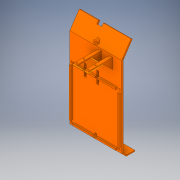
# Autodesk Inventor part: chassis-akksi-top
Saved by Autodesk Inventor 2019 (Build 230136000, 136)
## iProperties
Created: 2019-02-14
Part Number: chassis-akksi-top
Material: Generic
Document SubType Name: Modeling
Designer: izsoandras
Density: 1 g/cm^3
Appearance: Default
Author: izsoandras
Autodesk Inventor part; units mm, degrees
ref_plane "YZ Plane" through (0, 0, 0) normal (1, 0, 0) x (0, 1, 0)
ref_plane "XZ Plane" through (0, 0, 0) normal (0, 1, 0) x (-1, 0, 0)
ref_plane "XY Plane" through (0, 0, 0) normal (0, 0, 1) x (1, 0, 0)
sketch "Sketch1" plane through (0, 0, 0) normal (0, 0, 1) x (1, 0, 0)
  line L0 (59, 131.5) -> (-36.0094, 131.5)
  line L1 (-36.0094, 131.5) -> (-36.0094, -49.2144)
  line L2 (-36.0094, -49.2144) -> (59, -49.2144)
  line L3 (59, -49.2144) -> (59, 131.5)
  point P0 (0, 0)
  point P1 (-36, 131.5)
  point P2 (59.0094, -49.2144)
  constraints: 8 end point, 2 parallel, 1 horizontal, 1 perpendicular, 4 other
extrude "Extrusion1" add sketch "Sketch1" along normal blind 3
sketch "Sketch2" plane through (0, 0, 3) normal (0, 0, 1) x (1, 0, 0)
  line L0 (16.62, 69.08) -> (14.03, 69.08)
  line L1 (14.03, 69.08) -> (14.03, 48.08)
  line L2 (14.03, 48.08) -> (16.62, 48.08)
  line L3 (16.62, 48.08) -> (16.62, 69.08)
  line L4 (-6.41, 48.08) -> (-6.41, 69.08)
  line L5 (-6.41, 69.08) -> (-9, 69.08)
  line L6 (-9, 69.08) -> (-9, 48.08)
  line L7 (-9, 48.08) -> (-6.41, 48.08)
  line L8 (59, 131.5) -> (-36.0094, 131.5)
  line L9 (-36.0094, 131.5) -> (-36.0094, -49.2144)
  line L10 (-36.0094, -49.2144) -> (59, -49.2144)
  line L11 (59, -49.2144) -> (59, 131.5)
  line L12 (17.12, 69.58) -> (13.53, 69.58)
  line L13 (13.53, 69.58) -> (13.53, 47.58)
  line L14 (13.53, 47.58) -> (17.12, 47.58)
  line L15 (17.12, 47.58) -> (17.12, 69.58)
  line L16 (-5.91, 69.58) -> (-9.5, 69.58)
  line L17 (-9.5, 69.58) -> (-9.5, 47.58)
  line L18 (-9.5, 47.58) -> (-5.91, 47.58)
  line L19 (-5.91, 47.58) -> (-5.91, 69.58)
  circle A0 centre (55.5094, 59.3944) radius 1.5
  circle A1 centre (55.5094, -36.7144) radius 1.5
  circle A2 centre (-32.5094, -36.7144) radius 1.5
  circle A3 centre (-32.5094, 59.3944) radius 1.5
  point P0 (0, 0)
extrude "Extrusion2" cut sketch "Sketch2" against normal up to next contours L3 L2 L1 L0 | L7 L6 L5 L4 | L15 L14 L13 L12 | L19 L18 L17 L16 | A0 | A1 | A2 | A3
sketch "Sketch3" plane through (0, 0, 3) normal (0, 0, 1) x (1, 0, 0)
  line L0 (-34.195, 54.8944) -> (-31.195, 54.8944) projected
  line L1 (-31.195, 54.8944) -> (-31.195, -32.2144) projected
  line L2 (-31.195, -32.2144) -> (-34.195, -32.2144) projected
  line L3 (-34.195, -32.2144) -> (-34.195, 54.8944) projected
  line L4 (54.195, 54.8944) -> (57.195, 54.8944) projected
  line L5 (57.195, 54.8944) -> (57.195, -32.2144) projected
  line L6 (57.195, -32.2144) -> (54.195, -32.2144) projected
  line L7 (54.195, -32.2144) -> (54.195, 54.8944) projected
  line L8 (-28.0094, -35.4) -> (51.0094, -35.4) projected
  line L9 (51.0094, -35.4) -> (51.0094, -38.4) projected
  line L10 (51.0094, -38.4) -> (-28.0094, -38.4) projected
  line L11 (-28.0094, -38.4) -> (-28.0094, -35.4) projected
  line L12 (51.0094, 61.08) -> (51.0094, 58.08) projected
  line L13 (-28.0094, 58.08) -> (-28.0094, 61.08) projected
  line L14 (17.12, 47.58) -> (17.12, 69.58) projected
  line L15 (51.0094, 58.08) -> (17.12, 58.08)
  line L16 (17.12, 58.08) -> (17.12, 61.08)
  line L17 (17.12, 61.08) -> (51.0094, 61.08)
  line L18 (51.0094, 61.08) -> (51.0094, 58.08)
  line L19 (13.53, 47.58) -> (13.53, 69.58) projected
  line L20 (-5.91, 69.58) -> (-5.91, 47.58) projected
  line L21 (13.53, 58.08) -> (-5.91, 58.08)
  line L22 (-5.91, 58.08) -> (-5.91, 61.08)
  line L23 (-5.91, 61.08) -> (13.53, 61.08)
  line L24 (13.53, 61.08) -> (13.53, 58.08)
  line L25 (-9.5, 47.58) -> (-9.5, 69.58) projected
  line L26 (-28.0094, 58.08) -> (-9.5, 58.08)
  line L27 (-9.5, 58.08) -> (-9.5, 61.08)
  line L28 (-9.5, 61.08) -> (-28.0094, 61.08)
  line L29 (-28.0094, 61.08) -> (-28.0094, 58.08)
  point P0 (0, 0)
  constraints: 24 end point, 7 point on line, 6 parallel, 3 horizontal, 3 perpendicular
extrude "Extrusion3" add sketch "Sketch3" along normal blind 3
sketch "Sketch4" plane through (0, 0, 0) normal (0, 0, -1) x (-1, 0, 0)
  line L0 (16, 116.5) -> (36, 116.5) projected
  line L1 (36, 116.5) -> (36, -41.136) projected
  line L2 (36, -41.136) -> (16, -41.136) projected
  line L3 (16, -41.136) -> (16, 116.5) projected
  line L4 (-59, 116.5) -> (-39, 116.5) projected
  line L5 (-39, 116.5) -> (-39, -41.136) projected
  line L6 (-39, -41.136) -> (-59, -41.136) projected
  line L7 (-59, -41.136) -> (-59, 116.5) projected
  line L8 (14.5, -41.136) -> (17.5, -41.136)
  line L9 (17.5, -41.136) -> (17.5, 116.5)
  line L10 (17.5, 116.5) -> (14.5, 116.5)
  line L11 (14.5, 116.5) -> (14.5, -41.136)
  line L12 (-37.5, 116.5) -> (-40.5, 116.5)
  line L13 (-40.5, 116.5) -> (-40.5, -41.136)
  line L14 (-40.5, -41.136) -> (-37.5, -41.136)
  line L15 (-37.5, -41.136) -> (-37.5, 116.5)
  point P0 (0, 0)
  dimension "d13" = 1.5
  dimension "d14" = 1.5
  dimension "d15" = 1.5
  dimension "d16" = 1.5
  constraints: 16 end point, 4 parallel, 3 point on line, 2 horizontal, 2 perpendicular
  measures "d13" distance between parallel lines of L3 L11
  measures "d14" distance between parallel lines of L3 L9
  measures "d15" distance between parallel lines of L5 L15
  measures "d16" distance between parallel lines of L5 L13
extrude "Extrusion4" add sketch "Sketch4" along normal blind 6.7 contours L0 L9 L2 L3 | L3 L8 L11 L10 | L4 L5 L6 L13 | L12 L15 L14 L5
sketch "Sketch5" plane through (0, 0, 0) normal (0, 0, -1) x (-1, 0, 0)
  line L0 (-37, -32) -> (-37, 32) projected
  line L1 (9, 32) -> (9, -32) projected
  line L2 (14.5, 116.5) -> (14.5, -41.136) projected
  line L3 (-37, 24.2384) -> (14.5, 24.2384)
  line L4 (14.5, 24.2384) -> (14.5, 21.2384)
  line L5 (14.5, 21.2384) -> (-37, 21.2384)
  line L6 (-37, 21.2384) -> (-37, 24.2384)
  line L7 (-37.5, 116.5) -> (-37.5, -41.136) projected
  line L8 (14.5, -16.674) -> (-37.5, -16.674)
  line L9 (-37.5, -16.674) -> (-37.5, -19.674)
  line L10 (-37.5, -19.674) -> (14.5, -19.674)
  line L11 (14.5, -19.674) -> (14.5, -16.674)
  point P0 (0, 0)
  dimension "d20" = 3
  dimension "d21" = 3
  constraints: 16 end point, 4 parallel, 4 point on line, 2 horizontal, 2 perpendicular
  measures "d20" distance between parallel lines of L10 L8
  measures "d21" distance between parallel lines of L3 L5
extrude "Extrusion5" add sketch "Sketch5" along normal blind 1.7 contours L0 L3 L1 L5 | L8 L1 L10 L0 | L0 L10 L7 L8 | L1 L3 L2 L5 | L8 L2 L10 L1
sketch "Sketch6" plane through (-36.0094, -49.2144, 0) normal (-1, 0, 0) x (0, 0, 1)
  line L0 (-6.7, 165.7144) -> (-16.7, 180.7144) projected
  line L1 (-16.7, 180.7144) -> (-44.2, 151.5422) projected
  line L2 (-44.2, -0.2856) -> (-44.2, 151.5422) projected
  line L3 (-21.064, -0.2856) -> (-44.2, -0.2856) projected
  line L4 (-21.064, 1.7144) -> (-21.064, -0.2856) projected
  line L5 (-21.064, 1.7144) -> (-13.064, 1.7144) projected
  line L6 (-13.064, 1.7144) -> (-6.7, 8.0784) projected
  line L7 (-6.7, 165.7144) -> (-6.7, 8.0784) projected
  line L8 (0, 180.7144) -> (0, 0) projected
  line L9 (0, 0) -> (3, 0) projected
  line L10 (3, 180.7144) -> (3, 0) projected
  line L11 (0, 180.7144) -> (3, 180.7144) projected
  line L12 (-16.7, 180.7144) -> (0, 155.6644)
  line L13 (0, 155.6644) -> (2.4962, 157.3285)
  line L14 (2.4962, 157.3285) -> (-14.2038, 182.3785)
  line L15 (-14.2038, 182.3785) -> (-16.7, 180.7144)
  point P0 (0, 49.2144)
  dimension "d24" = 3
  dimension "d25" = 0
  constraints: 8 end point, 2 parallel, 1 perpendicular, 1 point on line
  measures "d24" distance between parallel lines of L0 L14
  measures "d25" distance from line of L8 L12.end
extrude "Extrusion6" add sketch "Sketch6" against normal blind 95 contours L0 L15 L14 L8 L12 | L8 L14 L13
sketch "Sketch7" plane through (-36.0094, -49.2144, 3) normal (-1, 0, 0) x (0, 0, 1)
  line L0 (-3, 165.7144) -> (-6.0944, 165.7144) projected
  line L1 (-6.0944, 165.7144) -> (0.2976, 156.1263)
  line L2 (-3, 161.0727) -> (-6.0944, 165.7144) projected
  line L3 (0.2976, 156.1263) -> (0.2976, 182.9184)
  line L4 (0, 0) -> (0, 180.7144) projected
  line L5 (0.2976, 182.9184) -> (-5.3952, 181.9603)
  line L6 (-5.3952, 181.9603) -> (-6.0944, 165.7144)
  point P0 (-3, 49.2144)
  constraints: 8 end point, 1 collinear, 1 parallel
extrude "Extrusion7" cut sketch "Sketch7" against normal blind 96
ref_plane "Work Plane1" through (16.62, 76.42, -7.3) normal (0, 1, 0) x (-1, 0, 0)
sketch "Sketch9" plane through (16.62, 76.42, -7.3) normal (0, 1, 0) x (-1, 0, 0)
  line L0 (0, 0) -> (8.7, 0) projected
  line L1 (8.7, 0) -> (8.7, -2.78) projected
  line L2 (16.62, -2.78) -> (8.7, -2.78) projected
  line L3 (16.62, 0) -> (16.62, -2.78) projected
  line L4 (16.62, 0) -> (25.62, 0) projected
  line L5 (25.62, 0) -> (25.62, 1.3) projected
  line L6 (0, 1.3) -> (25.62, 1.3) projected
  line L7 (0, 0) -> (0, 1.3) projected
  line L8 (8.2, -3.9038) -> (17.12, -3.9038)
  line L9 (17.12, -3.9038) -> (17.12, -9.4)
  line L10 (17.12, -9.4) -> (8.2, -9.4)
  line L11 (8.2, -9.4) -> (8.2, -3.9038)
  line L12 (52.6294, -6.9038) -> (52.6294, -9.4) projected
  line L13 (52.6294, -6.9038) -> (-42.3706, -6.9038) projected
  line L14 (-42.3706, -9.4) -> (-42.3706, -6.9038) projected
  line L15 (52.6294, -9.4) -> (-42.3706, -9.4) projected
  point P0 (16.62, 7.3)
  dimension "d35" = 0
  dimension "d36" = 3
  dimension "d37" = 0.5
  dimension "d38" = 0.5
  constraints: 8 end point, 2 parallel, 1 horizontal, 1 perpendicular
  measures "d35" distance between parallel lines of L15 L10
  measures "d36" distance between parallel lines of L13 L8
  measures "d37" distance between parallel lines of L1 L11
  measures "d38" distance between parallel lines of L9 L3
extrude "Extrusion8" cut sketch "Sketch9" along normal through all contours L8 L9 L13 L11 | L13 L9 L10 L11
sketch "Sketch10" plane through (0, 0, 3) normal (0, 0, 1) x (1, 0, 0)
  circle A0 centre (10.9691, 112.16) radius 1.5 projected
  circle A1 centre (11.8, -33.62) radius 2 projected
  circle A2 centre (10.9691, 112.16) radius 4 projected
  arc A3 (8.1427, -32) -> (9, -30.7634) centre (11.8, -33.62) ccw projected
  circle A4 centre (11.8, -33.62) radius 4
  point P0 (0, 0)
  constraints: 1 centre point, 1 coincident, 1 concentric
extrude "Extrusion9" cut sketch "Sketch10" along normal blind 3 contours A1 | A4 A3
sketch "Sketch11" plane through (0, 0, 3) normal (0, 0, 1) x (1, 0, 0)
  circle A0 centre (10.9691, 112.16) radius 4 projected
  circle A1 centre (10.9691, 112.16) radius 1.5 projected
  point P0 (0, 0)
extrude "Extrusion10" add sketch "Sketch11" against normal blind 9.75 contours A0 | A1
sketch "Sketch12" plane through (10.9691, 112.16, 3) normal (0, 0, 1) x (1, 0, 0)
  circle A0 centre (0, 0) radius 4
  circle A1 centre (0, 0) radius 1.5 projected
  point P0 (-10.9691, -112.16)
  constraints: 1 centre point
extrude "Extrusion11" cut sketch "Sketch12" against normal up to next contours A1
sketch "Sketch13" plane through (0, 0, 3) normal (0, 0, 1) x (1, 0, 0)
  circle A0 centre (11.8, -33.62) radius 2 projected
  point P0 (0, 0)
extrude "Extrusion12" cut sketch "Sketch13" against normal up to next
sketch "Sketch15" plane through (59, -49.2144, 0) normal (1, 0, 0) x (0, 0, -1)
  line L0 (44.2, 151.5422) -> (16.7, 180.7144) projected
  line L1 (16.7, 180.7144) -> (6.7, 165.7144) projected
  line L2 (6.7, 8.0784) -> (6.7, 165.7144) projected
  line L3 (6.7, 8.0784) -> (13.064, 1.7144) projected
  line L4 (21.064, 1.7144) -> (13.064, 1.7144) projected
  line L5 (21.064, 1.7144) -> (21.064, -0.2856) projected
  line L6 (44.2, -0.2856) -> (21.064, -0.2856) projected
  line L7 (44.2, 151.5422) -> (44.2, -0.2856) projected
  line L8 (0, 8.0784) -> (0, 155.6644) projected
  line L9 (-3.0214, 8.0784) -> (0, 8.0784)
  line L10 (0, 8.0784) -> (6.364, 1.7144)
  line L11 (6.364, 1.7144) -> (21.064, 1.7144)
  line L12 (21.064, -0.2856) -> (5.4901, -0.2856)
  line L13 (5.4901, -0.2856) -> (-2.8739, 8.0784)
  point P0 (0, 49.2144)
  dimension "d51" = 135
  dimension "d52" = 45
  constraints: 10 end point, 2 horizontal, 1 collinear, 1 point on line
  measures "d51" angle of L9 L10
  measures "d52" angle of L9 L13
extrude "Extrusion13" add sketch "Sketch15" against normal blind 95 contours L12 L13 L9 L10 L11 L4 L5
sketch "Sketch16" plane through (40.5, -41.136, -6.7) normal (1, 0, 0) x (0, 0, -1)
  line L0 (-6.7, 0) -> (-6.7, 152.9944) projected
  line L1 (-6.7, 152.9944) -> (-9.7, 148.4944) projected
  line L2 (-9.7, -8.0784) -> (-9.7, 148.4944) projected
  line L3 (-6.7, -8.0784) -> (-9.7, -8.0784) projected
  line L4 (-6.7, -8.0784) -> (-6.7, -2.8739) projected
  line L5 (-6.7, -2.8739) -> (-1.2099, -8.364) projected
  line L6 (-1.2099, -8.364) -> (14.364, -8.364) projected
  line L7 (14.364, -8.364) -> (14.364, -6.364) projected
  line L8 (14.364, -6.364) -> (-0.336, -6.364) projected
  line L9 (-0.336, -6.364) -> (-6.7, 0) projected
  line L10 (-6.7, 0) -> (0, 0) projected
  line L11 (0, 0) -> (6.364, -6.364)
  line L12 (14.364, -6.364) -> (-0.336, -6.364) projected
  line L13 (-0.336, -6.364) -> (-6.7, 0)
  point P0 (-6.7, 41.136)
  constraints: 4 end point, 1 collinear, 1 point on line
extrude "Extrusion14" add sketch "Sketch16" against normal blind 3 contours L10 L11 L8 L9
sketch "Sketch17" plane through (-17.5, -41.136, -6.7) normal (-1, 0, 0) x (0, 0, 1)
  line L0 (6.7, 147.586) -> (0, 157.636) projected
  line L1 (0, 0) -> (0, 157.636) projected
  line L2 (0, 0) -> (-6.364, -6.364) projected
  line L3 (0.336, -6.364) -> (-6.364, -6.364) projected
  line L4 (6.7, 0) -> (0.336, -6.364) projected
  line L5 (6.7, 21.462) -> (6.7, 0) projected
  line L6 (6.7, 21.462) -> (5, 21.462) projected
  line L7 (5, 21.462) -> (5, 24.462) projected
  line L8 (5, 24.462) -> (6.7, 24.462) projected
  line L9 (6.7, 147.586) -> (6.7, 24.462) projected
  line L10 (-6.364, -6.364) -> (0, 0) projected
  line L11 (0, 0) -> (-6.364, -6.364)
  line L12 (-6.364, -6.364) -> (0.336, -6.364) projected
  line L13 (-6.364, -6.364) -> (0.336, -6.364)
  line L14 (0.336, -6.364) -> (6.7, 0) projected
  line L15 (0.336, -6.364) -> (6.7, 0)
  line L16 (6.7, 0) -> (0, 0)
  point P0 (6.7, 41.136)
  constraints: 8 end point, 3 collinear, 1 perpendicular
extrude "Extrusion15" add sketch "Sketch17" against normal blind 3 contours L16 L4 L3 L2
sketch "Sketch18" plane through (59, -49.5, -21.064) normal (0, -1, 0) x (1, 0, 0)
  line L0 (-34, 0) -> (-26, 0) projected
  line L1 (-26, 0) -> (-26, 9.364) projected
  line L2 (-34, 9.364) -> (-26, 9.364) projected
  line L3 (-34, 0) -> (-34, 9.364) projected
  point P0 (-59, 21.064)
extrude "Extrusion16" cut sketch "Sketch18" against normal up to next
sketch "Sketch19" plane through (59, -49.2144, 3) normal (1, 0, 0) x (0, 0, -1)
  line L0 (3, 0) -> (3, 5.2045) projected
  line L1 (3, 5.2045) -> (0, 8.2045)
  line L2 (0, 0) -> (0, 156.5727) projected
  line L3 (3, 0) -> (0, 0) projected
  line L4 (0, 0) -> (3, 0)
  line L5 (3, 8.0784) -> (3, 5.2045) projected
  line L6 (3, 0) -> (3, 5.2045)
  point P0 (3, 49.2144)
  dimension "d61" = 45
  constraints: 6 end point, 1 collinear, 1 perpendicular, 1 point on line
  measures "d61" angle of L1 L0
extrude "Extrusion17" cut sketch "Sketch19" against normal through all
ref_plane "Work Plane2" through (29.2806, 102.08, 35) normal (0, 1, 0) x (-1, 0, 0)
sketch "Sketch20" plane through (29.2806, 102.08, 35) normal (0, 1, 0) x (-1, 0, 0)
  line L0 (-4.6, -7) -> (-4.6, 1) projected
  line L1 (-4.6, 1) -> (-5.4, 1) projected
  line L2 (-5.4, 1) -> (-5.4, 9) projected
  line L3 (-5.4, 9) -> (3.6, 9) projected
  line L4 (3.6, 9) -> (3.6, 2) projected
  line L5 (3.6, 2) -> (4.4, 2) projected
  line L6 (4.4, 2) -> (4.4, -7) projected
  line L7 (4.4, -7) -> (-4.6, -7) projected
  circle A0 centre (10.4, -3.2) radius 1.2 projected
  circle A1 centre (-10.4, 9.8) radius 1.2 projected
  circle A2 centre (10.4, 9.8) radius 1.2 projected
  circle A3 centre (-10.4, -3.2) radius 1.2 projected
  line L8 (10.6, 12) -> (-10.6, 12) projected
  arc A4 (-10.6, 12) -> (-12.6, 10) centre (-10.6, 10) ccw projected
  line L9 (-12.6, 10) -> (-12.6, -10) projected
  arc A5 (-12.6, -10) -> (-10.6, -12) centre (-10.6, -10) ccw projected
  line L10 (-10.6, -12) -> (10.6, -12) projected
  arc A6 (10.6, -12) -> (12.6, -10) centre (10.6, -10) ccw projected
  line L11 (12.6, -10) -> (12.6, 10) projected
  arc A7 (12.6, 10) -> (10.6, 12) centre (10.6, 10) ccw projected
  line L12 (-13.4, 12.8) -> (-7.4, 12.8)
  line L13 (-7.4, 12.8) -> (-7.4, -32)
  line L14 (-7.4, -32) -> (-13.4, -32)
  line L15 (-13.4, -32) -> (-13.4, 12.8)
  line L16 (-29.7194, -32) -> (65.29, -32) projected
  line L17 (7.4, 12.8) -> (13.4, 12.8)
  line L18 (13.4, 12.8) -> (13.4, -32)
  line L19 (13.4, -32) -> (7.4, -32)
  line L20 (7.4, -32) -> (7.4, 12.8)
  point P0 (29.2806, -35)
  dimension "d67" = 3
  dimension "d68" = 3
  dimension "d69" = 3
  dimension "d70" = 0
  dimension "d79" = 3
  dimension "d80" = 3
  dimension "d81" = 3
  dimension "d82" = 0
  constraints: 16 end point, 4 parallel, 2 horizontal, 2 perpendicular
  measures "d67" distance from line of L15 A1.centre
  measures "d68" distance from line of L13 A1.centre
  measures "d69" distance from line of L12 A1.centre
  measures "d70" distance between parallel lines of L16 L14
  measures "d79" distance from line of L17 A2.centre
  measures "d80" distance from line of L18 A2.centre
  measures "d81" distance from line of L20 A2.centre
  measures "d82" distance between parallel lines of L16 L19
extrude "Extrusion18" add sketch "Sketch20" along normal blind 2 contours A7 L11 A6 L10 L20 L8 | L8 L20 L17 L18 L16 L10 A6 L11 A7 | L13 L10 A5 L9 A4 L8 | L8 A4 L9 A5 L10 L13 L14 L15 L12
sketch "Sketch21" plane through (29.2806, 102.08, 35) normal (0, -1, 0) x (1, 0, 0)
  line L0 (13.4, 12.8) -> (13.4, -32) projected
  line L1 (7.4, -14.5) -> (13.4, -14.5)
  line L2 (13.4, -14.5) -> (13.4, -32)
  line L3 (13.4, -32) -> (7.4, -32)
  line L4 (7.4, -32) -> (7.4, -14.5)
  line L5 (-65.29, -32) -> (29.7194, -32) projected
  line L6 (7.4, 12.8) -> (7.4, -32) projected
  line L7 (-13.4, -32) -> (-13.4, 12.8) projected
  line L8 (21.7288, -32) -> (-57.29, -32) projected
  line L9 (-13.4, -14.5) -> (-7.4, -14.5)
  line L10 (-7.4, -14.5) -> (-7.4, -32)
  line L11 (-7.4, -32) -> (-13.4, -32)
  line L12 (-13.4, -32) -> (-13.4, -14.5)
  line L13 (-7.4, -32) -> (-7.4, 12.8) projected
  point P0 (-29.2806, -35)
  dimension "d73" = 0
  dimension "d74" = 0
  dimension "d83" = 0
  dimension "d84" = 17.5
  dimension "d85" = 17.5
  constraints: 16 end point, 4 parallel, 3 point on line, 2 horizontal, 2 perpendicular
  measures "d73" distance between parallel lines of L5 L3
  measures "d74" distance between parallel lines of L6 L4
  measures "d83" distance between parallel lines of L13 L10
  measures "d84" distance of L9.end L10.end
  measures "d85" distance of L1.end L2.end
extrude "Extrusion19" add sketch "Sketch21" along normal blind 17.5
sketch "Sketch22" plane through (42.6806, 102.08, 47.8) normal (1, 0, 0) x (0, 0, -1)
  line L0 (44.8, -17.5) -> (27.3, -17.5) projected
  line L1 (27.3, -17.5) -> (44.8, -17.5)
  line L2 (27.3, 0) -> (27.3, -17.5) projected
  line L3 (44.8, -17.5) -> (27.3, 0)
  line L4 (27.3, 0) -> (27.3, -17.5)
  point P0 (47.8, -102.08)
  constraints: 6 end point, 2 collinear
extrude "Extrusion20" cut sketch "Sketch22" against normal through all
equation "\"d14\" = d13"
equation "\"d15\" = d13"
equation "\"d16\" = d13"
equation "\"d68\" = d67"
equation "\"d69\" = d67"
equation "\"d79\" = d67"
equation "\"d80\" = d79"
equation "\"d81\" = d79"
body "Solid1"
